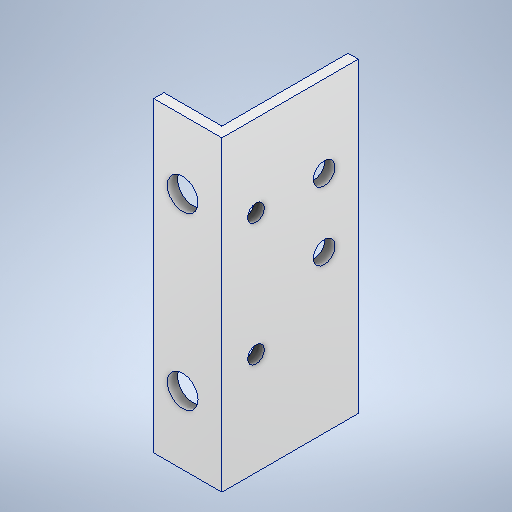
# Autodesk Inventor part: x_bracket
Saved by Autodesk Inventor 2025 (Build 290162000, 162)
## iProperties
Created: 2024-04-25
Part Number: x_bracket
Material: Hliník 6061
Document SubType Name: Modeling
Designer: rader
Density: 2.7 g/cm^3
Appearance: Hliník – plochý
Author: rader
Autodesk Inventor part; units mm, degrees
ref_plane "YZ Plane" through (0, 0, 0) normal (1, 0, 0) x (0, 1, 0)
ref_plane "XZ Plane" through (0, 0, 0) normal (0, 1, 0) x (-1, 0, 0)
ref_plane "XY Plane" through (0, 0, 0) normal (0, 0, 1) x (1, 0, 0)
sketch "Náčrt1" plane through (0, 0, 0) normal (0, 0, 1) x (1, 0, 0)
  line L0 (-10, 0) -> (0, 0)
  line L1 (0, 0) -> (0, 20)
  line L2 (0, 20) -> (-1.5, 20)
  line L3 (-1.5, 20) -> (-1.5, 1.5)
  line L4 (-1.5, 1.5) -> (-10, 1.5)
  line L5 (-10, 1.5) -> (-10, 0)
  line L6 (-12, 0) -> (2, 0) projected
  line L7 (0, 24) -> (0, -4) projected
  point P0 (0, 0)
  dimension "d0" = 20
  dimension "d1" = 10
  dimension "d2" = 1.5
  dimension "d3" = 1.5
  constraints: 12 end point, 5 perpendicular, 3 collinear, 1 horizontal
  measures "d0" distance of L0.end L1.end
  measures "d1" distance of L0.start L0.end
  measures "d2" distance between parallel lines of L3 L1
  measures "d3" distance between parallel lines of L4 L0
extrude "Vysunutí1" add sketch "Náčrt1" along normal mid plane 45
sketch "Náčrt2" plane through (-10, 1.5, 22.5) normal (0, 1, 0) x (1, 0, 0)
  line L0 (0, 0) -> (0, 45) projected
  line L1 (8.5, 0) -> (0, 0) projected
  line L2 (8.5, 45) -> (8.5, 0) projected
  line L3 (0, 45) -> (8.5, 45) projected
  point P0 (10, 22.5)
  point P1 (4.25, 35)
  point P2 (4.25, 10)
  point P3 (4.25, 0)
  dimension "d6" = 4.25
  dimension "d7" = 4.25
  dimension "d8" = 25
  dimension "d9" = 10
  constraints: 1 midpoint
  measures "d6" distance from line of L0 point (4.25, 10)
  measures "d7" distance from line of L0 point (4.25, 35)
  measures "d8" distance of point (4.25, 10) point (4.25, 35)
  measures "d9" distance of point (4.25, 0) point (4.25, 10)
hole "Díra1" at (-5.75, 1.5, -12.5) at (-5.75, 1.5, 12.5) direction (0, -1, 0) diameter 4.5 end through all
sketch "Náčrt3" plane through (-1.5, 1.5, 22.5) normal (-1, 0, 0) x (0, 0, 1)
  line L0 (-45, 0) -> (0, 0) projected
  line L1 (0, 18.5) -> (0, 0) projected
  line L2 (-45, 18.5) -> (0, 18.5) projected
  line L3 (-45, 0) -> (-45, 18.5) projected
  point P0 (-22.5, -1.5)
  point P1 (-12, 13.5)
  point P2 (-22, 13.5)
  dimension "d17" = 10
  dimension "d18" = 5
  dimension "d19" = 5
  dimension "d20" = 12
  measures "d17" distance of point (-22, 13.5) point (-12, 13.5)
  measures "d18" distance from line of L2 point (-12, 13.5)
  measures "d19" distance from line of L2 point (-22, 13.5)
  measures "d20" distance from line of L1 point (-12, 13.5)
hole "Díra2" at (-1.5, 15, 10.5) at (-1.5, 15, 0.5) direction (1, 0, 0) diameter 3.2 end through all
sketch "Náčrt4" plane through (-1.5, 1.5, 22.5) normal (-1, 0, 0) x (0, 0, 1)
  circle A0 centre (-22, 13.5) radius 1.6 projected
  circle A1 centre (-12, 13.5) radius 1.6 projected
  line L0 (-45, 0) -> (0, 0) projected
  line L1 (0, 18.5) -> (0, 0) projected
  line L2 (-45, 18.5) -> (0, 18.5) projected
  line L3 (-45, 0) -> (-45, 18.5) projected
  line L4 (-45, -1.5) -> (0, -1.5) projected
  point P0 (-22.5, -1.5)
  point P1 (-30, 3.5)
  point P2 (-12, 3.5)
  dimension "d28" = 5
  dimension "d29" = 5
  dimension "d30" = 18
  dimension "d31" = 12
  measures "d28" distance from line of point (-12, 3.5) L4
  measures "d29" distance from line of point (-30, 3.5) L4
  measures "d30" distance of point (-30, 3.5) point (-12, 3.5)
  measures "d31" distance from line of L1 point (-12, 3.5)
hole "Díra3" at (-1.5, 5, -7.5) at (-1.5, 5, 10.5) direction (1, 0, 0) diameter 2.459 end through all thread size "M3x0.5" class "6H" standard "ISO Metric profile"
